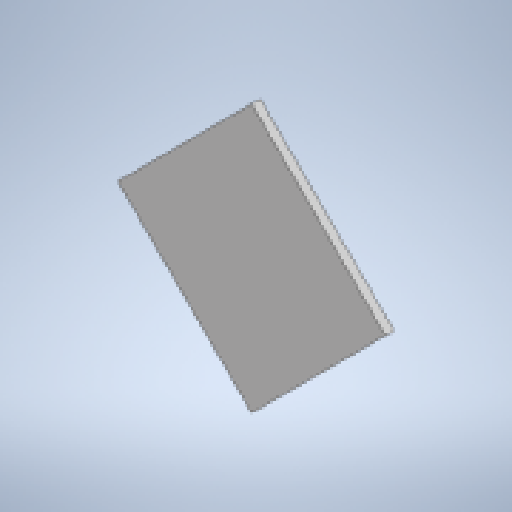
# Autodesk Inventor part: Template220
Saved by Autodesk Inventor 2025.1 (Build 291241000, 241)
## iProperties
Created: 2025-05-09
Part Number: Template220
Material: Generic
Document SubType Name: Modeling
Designer: User
Density: 1 g/cm^3
Appearance: Default
Author: User
Autodesk Inventor part; units mm, degrees
ref_plane "YZ Plane" through (0, 0, 0) normal (1, 0, 0) x (0, 1, 0)
ref_plane "XZ Plane" through (0, 0, 0) normal (0, 1, 0) x (-1, 0, 0)
ref_plane "XY Plane" through (0, 0, 0) normal (0, 0, 1) x (1, 0, 0)
sketch "Sketch1" plane through (0, 0, 0) normal (0, 0, 1) x (1, 0, 0)
  line L0 (-46.0933, 91.1044) -> (-62.0933, 91.1044) projected
  line L1 (-54.0933, 118.5442) -> (-209.6568, -37.0193)
  line L2 (-209.6568, -37.0193) -> (-54.0933, -192.5828)
  line L3 (-54.0933, -192.5828) -> (101.4702, -37.0193)
  line L4 (101.4702, -37.0193) -> (-54.0933, 118.5442)
  line L5 (-54.0933, 91.1044) -> (165.9067, 91.1044) construction
  line L6 (-25.3821, 79.8544) -> (-25.3821, 89.8544)
  line L7 (-82.7831, 89.8544) -> (-82.7831, 79.8544) projected
  line L8 (-54.0933, 91.1044) -> (-54.0933, 151.1044)
  line L9 (-82.7831, 89.8544) -> (-54.0933, 118.5442)
  line L10 (-82.7831, 89.8544) -> (-42.2096, 89.8544) construction
  point P0 (0, 0)
  dimension "d0" = 220
  dimension "d1" = 135
  dimension "d2" = 220
  dimension "d3" = 60
  dimension "d4" = 45
  constraints: 18 end point, 2 equal length, 2 horizontal, 2 parallel, 2 perpendicular, 1 point on line, 1 vertical, 2 other
  measures "d0" distance of L1.start L1.end
  measures "d1" angle of L1 L5
  measures "d2" distance of L2.end L1.end
  measures "d3" distance of L8.start L8.end
  measures "d4" angle of L10 L9
extrude "Extrusion1" add sketch "Sketch1" along normal blind 10
sketch "Sketch2" plane through (0, 0, 0) normal (0, 0, -1) x (-1, 0, 0)
  line L0 (209.6568, -37.0193) -> (54.0933, -192.5828) projected
  line L1 (54.0933, 118.5442) -> (209.6568, -37.0193) projected
  line L2 (-101.4702, -37.0193) -> (54.0933, 118.5442) projected
  line L3 (54.0933, -192.5828) -> (-101.4702, -37.0193) projected
  line L4 (-101.4702, -37.0193) -> (209.6568, -37.0193)
  line L5 (54.0933, -192.5828) -> (54.0933, 118.5442)
  line L6 (74.0933, -3.2956) -> (34.0933, -3.2956) projected
  line L7 (34.0933, 39.0692) -> (74.0933, 39.0692)
  line L8 (74.0933, 39.0692) -> (74.0933, -3.2956)
  line L9 (74.0933, -3.2956) -> (34.0933, -3.2956)
  line L10 (34.0933, -3.2956) -> (34.0933, 39.0692)
  point P0 (0, 0)
  constraints: 12 end point, 2 horizontal, 2 parallel, 2 perpendicular
sketch "Sketch3" plane through (0, 0, 0) normal (0, 0, -1) x (-1, 0, 0)
  line L0 (-101.4702, -37.0193) -> (209.6568, -37.0193) projected
  line L1 (54.0933, -192.5828) -> (54.0933, 118.5442) projected
  circle A0 centre (54.0933, -37.0193) radius 15.2178
  point P0 (0, 0)
  constraints: 1 centre point, 1 midpoint
extrude "Extrusion2" cut sketch "Sketch3" against normal blind 10
body "Solid1"
